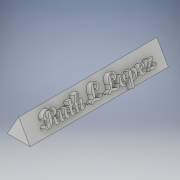
# Autodesk Inventor part: namePlateV01
Saved by Autodesk Inventor 2018.2 (Build 222227000, 227)
## iProperties
Created: 2018-02-15
Part Number: namePlateV01
Material: Generic
Document SubType Name: Modeling
Designer: steele
Density: 1 g/cm^3
Appearance: Default
Author: steele
Autodesk Inventor part; units mm, degrees
ref_plane "YZ Plane" through (0, 0, 0) normal (1, 0, 0) x (0, 1, 0)
ref_plane "XZ Plane" through (0, 0, 0) normal (0, 1, 0) x (-1, 0, 0)
ref_plane "XY Plane" through (0, 0, 0) normal (0, 0, 1) x (1, 0, 0)
sketch "Sketch1" plane through (0, 0, 0) normal (0, 0, 1) x (1, 0, 0)
  line L0 (0, 0) -> (12.7, 0)
  line L1 (0, 0) -> (0, 34.2679) construction
  line L2 (0, 21.997) -> (12.7, 0)
  line L3 (0, 0) -> (-12.7, 0)
  line L4 (0, 21.997) -> (-12.7, 0)
  dimension "d0" = 12.7
  dimension "d1" = 25.4
  constraints: 10 end point, 1 horizontal, 1 point on line, 1 symmetric about line, 1 vertical
  measures "d0" distance of L0.start L0.end
  measures "d1" distance of L2.start L0.end
extrude "Extrusion1" add sketch "Sketch1" along normal mid plane 152.4
sketch "Sketch2" plane through (0, 21.997, 76.2) normal (0.866, 0.5, 0) x (0, 0, -1)
  line L0 (0, -25.4) -> (0, 0) construction
  line L1 (152.4, -12.7) -> (0, -12.7) construction
  line L2 (0, -12.7) -> (152.4, -12.7) construction
  spline S0 degree 2 poles (32.3187, -16.7248) (31.0929, -18.0517) (29.1594, -19.2901) (28.1611, -19.2901) knots 0 0 0 1 2 2 2
  spline S1 degree 2 poles (28.1611, -19.2901) (27.1376, -19.2901) (25.8865, -17.9506) (25.8865, -16.8638) knots 0 0 0 1 2 2 2
  spline S2 degree 2 poles (25.8865, -16.8638) (25.8865, -16.2067) (26.4804, -13.9321) (26.4804, -13.3255) knots 0 0 0 1 2 2 2
  spline S3 degree 2 poles (26.4804, -13.3255) (26.4804, -12.3399) (25.8486, -12.3146) knots 0 0 0 1 1 1
  spline S4 degree 2 poles (25.8486, -12.3146) (25.4569, -12.2893) (25.4569, -11.9481) knots 0 0 0 1 1 1
  spline S5 degree 2 poles (25.4569, -11.9481) (25.4569, -11.3289) (25.9118, -11.3289) knots 0 0 0 1 1 1
  line L3 (25.9118, -11.3289) -> (26.6068, -11.3668)
  spline S6 degree 2 poles (26.6068, -11.3668) (27.6051, -11.3668) (28.7677, -9.4334) (28.7677, -8.0686) knots 0 0 0 1 2 2 2
  spline S7 degree 2 poles (28.7677, -8.0686) (28.7677, -4.8968) (25.1536, -4.8968) knots 0 0 0 1 1 1
  spline S8 degree 2 poles (25.1536, -4.8968) (22.8537, -4.8968) (19.2901, -7.3862) (19.2901, -8.9153) knots 0 0 0 1 2 2 2
  spline S9 degree 2 poles (19.2901, -8.9153) (19.2901, -9.7746) (20.1494, -10.2169) knots 0 0 0 1 1 1
  spline S10 degree 2 poles (20.1494, -10.2169) (20.5538, -10.4317) (20.5538, -10.735) knots 0 0 0 1 1 1
  spline S11 degree 2 poles (20.5538, -10.735) (20.5538, -11.0003) (18.9615, -11.708) (18.6709, -11.708) knots 0 0 0 1 2 2 2
  spline S12 degree 2 poles (18.6709, -11.708) (18.2033, -11.708) (17.4578, -10.5075) (17.4578, -9.724) knots 0 0 0 1 2 2 2
  spline S13 degree 2 poles (17.4578, -9.724) (17.4578, -7.3989) (22.1839, -4.088) (25.5832, -4.088) knots 0 0 0 1 2 2 2
  spline S14 degree 2 poles (25.5832, -4.088) (28.4391, -4.088) (31.6236, -6.5396) (31.6236, -8.2961) knots 0 0 0 1 2 2 2
  spline S15 degree 2 poles (31.6236, -8.2961) (31.6236, -9.3955) (29.8671, -11.4679) (27.3018, -12.0492) knots 0 0 0 1 2 2 2
  spline S16 degree 2 poles (27.3018, -12.0492) (28.237, -12.58) (29.0836, -13.831) (29.0836, -14.7788) knots 0 0 0 1 2 2 2
  spline S17 degree 2 poles (29.0836, -14.7788) (29.0836, -15.2969) (28.8688, -16.5985) (28.8688, -16.7754) knots 0 0 0 1 2 2 2
  spline S18 degree 2 poles (28.8688, -16.7754) (28.8688, -17.6726) (29.5891, -17.6726) knots 0 0 0 1 1 1
  spline S19 degree 2 poles (29.5891, -17.6726) (30.5369, -17.6726) (32.3187, -15.5117) knots 0 0 0 1 1 1
  line L4 (32.3187, -15.5117) -> (32.3187, -16.7248)
  spline S20 degree 2 poles (26.9227, -6.7038) (26.0634, -7.3989) (25.4821, -8.9911) (24.8882, -13.2623) (24.1426, -15.7897) (22.2977, -18.0264) (19.6818, -19.2901) (18.2791, -19.2901) knots 0 0 0 1 2 3 4 5 6 6 6
  spline S21 degree 2 poles (18.2791, -19.2901) (16.7754, -19.2901) (15.2716, -17.8242) (15.2716, -16.8765) knots 0 0 0 1 2 2 2
  spline S22 degree 2 poles (15.2716, -16.8765) (15.2716, -16.5732) (15.7391, -16.0803) (17.205, -15.2463) (17.483, -15.2463) knots 0 0 0 1 2 3 3 3
  spline S23 degree 2 poles (17.483, -15.2463) (17.8242, -15.2463) (17.8242, -15.6507) knots 0 0 0 1 1 1
  spline S24 degree 2 poles (17.8242, -15.6507) (17.8242, -15.7392) (17.6094, -16.9776) (17.6094, -17.1039) knots 0 0 0 1 2 2 2
  spline S25 degree 2 poles (17.6094, -17.1039) (17.6094, -17.6852) (18.2791, -18.4561) (18.7973, -18.4561) knots 0 0 0 1 2 2 2
  spline S26 degree 2 poles (18.7973, -18.4561) (19.884, -18.4561) (21.5647, -15.6886) (22.2471, -10.28) (23.3591, -7.8411) (25.4948, -6.35) (26.3414, -6.35) knots 0 0 0 1 2 3 4 5 5 5
  spline S27 degree 2 poles (26.3414, -6.35) (26.5815, -6.35) (26.9227, -6.7038) knots 0 0 0 1 1 1
  spline S28 degree 2 poles (43.5149, -16.7375) (42.1248, -18.0391) (40.2672, -19.2901) (39.5216, -19.2901) knots 0 0 0 1 2 2 2
  spline S29 degree 2 poles (39.5216, -19.2901) (38.6876, -19.2901) (37.803, -17.9632) (37.803, -16.8386) knots 0 0 0 1 2 2 2
  spline S30 degree 2 poles (37.803, -16.8386) (36.6404, -18.1022) (34.8207, -19.3154) (33.9488, -19.3154) knots 0 0 0 1 2 2 2
  spline S31 degree 2 poles (33.9488, -19.3154) (33.14, -19.3154) (32.1796, -17.9885) (32.1796, -16.8638) knots 0 0 0 1 2 2 2
  spline S32 degree 2 poles (32.1796, -16.8638) (32.1796, -14.6777) (33.6455, -10.7097) knots 0 0 0 1 1 1
  line L5 (33.6455, -10.7097) -> (36.4635, -10.1537)
  spline S33 degree 2 poles (36.4635, -10.1537) (34.7196, -15.1831) (34.7196, -16.6111) knots 0 0 0 1 1 1
  spline S34 degree 2 poles (34.7196, -16.6111) (34.7196, -17.6094) (35.4779, -17.6094) knots 0 0 0 1 1 1
  spline S35 degree 2 poles (35.4779, -17.6094) (36.0212, -17.6094) (37.6388, -15.8402) (37.8409, -15.1831) knots 0 0 0 1 2 2 2
  line L6 (37.8409, -15.1831) -> (39.2184, -10.7097)
  line L7 (39.2184, -10.7097) -> (42.0869, -10.1284)
  spline S36 degree 2 poles (42.0869, -10.1284) (41.0886, -13.2876) (40.343, -15.8529) (40.343, -16.3584) knots 0 0 0 1 2 2 2
  spline S37 degree 2 poles (40.343, -16.3584) (40.343, -17.344) (41.0128, -17.344) knots 0 0 0 1 1 1
  spline S38 degree 2 poles (41.0128, -17.344) (41.5688, -17.344) (42.6303, -16.3457) knots 0 0 0 1 1 1
  line L8 (42.6303, -16.3457) -> (43.5149, -15.5243)
  line L9 (43.5149, -15.5243) -> (43.5149, -16.7375)
  spline S39 degree 2 poles (49.6943, -16.7375) (48.3674, -18.0391) (46.434, -19.2901) (45.562, -19.2901) knots 0 0 0 1 2 2 2
  spline S40 degree 2 poles (45.562, -19.2901) (44.6648, -19.2901) (43.5401, -17.7737) (43.5401, -16.5353) knots 0 0 0 1 2 2 2
  spline S41 degree 2 poles (43.5401, -16.5353) (43.5401, -15.4359) (44.0835, -13.6541) knots 0 0 0 1 1 1
  line L10 (44.0835, -13.6541) -> (44.5258, -12.0618)
  line L11 (44.5258, -12.0618) -> (43.7171, -12.0998)
  line L12 (43.7171, -12.0998) -> (44.0583, -10.457)
  line L13 (44.0583, -10.457) -> (45.0566, -10.4191)
  line L14 (45.0566, -10.4191) -> (46.0422, -7.1461)
  line L15 (46.0422, -7.1461) -> (48.8476, -6.5648)
  line L16 (48.8476, -6.5648) -> (47.7608, -10.2169)
  line L17 (47.7608, -10.2169) -> (49.2393, -10.1284)
  line L18 (49.2393, -10.1284) -> (48.8982, -11.7459)
  line L19 (48.8982, -11.7459) -> (47.268, -11.8723)
  line L20 (47.268, -11.8723) -> (46.5603, -14.2227)
  spline S42 degree 2 poles (46.5603, -14.2227) (46.2065, -15.4485) (46.2065, -16.1688) knots 0 0 0 1 1 1
  spline S43 degree 2 poles (46.2065, -16.1688) (46.2065, -16.6616) (46.6993, -17.2808) (47.0911, -17.2808) knots 0 0 0 1 2 2 2
  spline S44 degree 2 poles (47.0911, -17.2808) (47.6218, -17.2808) (48.6707, -16.5985) (49.6943, -15.5243) knots 0 0 0 1 2 2 2
  line L21 (49.6943, -15.5243) -> (49.6943, -16.7375)
  spline S45 degree 2 poles (60.107, -16.7375) (57.6176, -19.3154) (56.0127, -19.3154) knots 0 0 0 1 1 1
  spline S46 degree 2 poles (56.0127, -19.3154) (55.305, -19.3154) (54.3699, -18.3423) (54.3699, -17.5968) knots 0 0 0 1 2 2 2
  spline S47 degree 2 poles (54.3699, -17.5968) (54.3699, -16.3331) (55.3303, -14.0458) knots 0 0 0 1 1 1
  spline S48 degree 2 poles (55.3303, -14.0458) (55.8484, -12.8074) (55.8484, -12.4283) knots 0 0 0 1 1 1
  spline S49 degree 2 poles (55.8484, -12.4283) (55.8484, -11.9987) (55.444, -11.9987) knots 0 0 0 1 1 1
  spline S50 degree 2 poles (55.444, -11.9987) (55.0144, -11.9987) (53.4221, -13.136) (52.5376, -14.1216) knots 0 0 0 1 2 2 2
  spline S51 degree 2 poles (52.5376, -14.1216) (52.1711, -16.0551) (52.1711, -18.772) knots 0 0 0 1 1 1
  line L22 (52.1711, -18.772) -> (49.8333, -19.3154)
  spline S52 degree 2 poles (49.8333, -19.3154) (49.6943, -18.216) (49.6943, -16.927) knots 0 0 0 1 1 1
  spline S53 degree 2 poles (49.6943, -16.927) (49.6943, -13.7931) (51.4129, -8.3972) (53.2579, -5.377) knots 0 0 0 1 2 2 2
  spline S54 degree 2 poles (53.2579, -5.377) (54.6353, -4.8209) (56.6824, -4.1133) (56.8214, -4.1133) knots 0 0 0 1 2 2 2
  spline S55 degree 2 poles (56.8214, -4.1133) (57.0994, -4.1133) (57.4786, -4.9979) (57.4786, -5.655) knots 0 0 0 1 2 2 2
  spline S56 degree 2 poles (57.4786, -5.655) (57.4786, -6.767) (56.1138, -9.4713) (54.6605, -11.3795) knots 0 0 0 1 2 2 2
  spline S57 degree 2 poles (54.6605, -11.3795) (56.0632, -10.5707) (56.9857, -10.1537) (57.4786, -10.1537) knots 0 0 0 1 2 2 2
  spline S58 degree 2 poles (57.4786, -10.1537) (58.0093, -10.1537) (58.6791, -10.9245) (58.6791, -11.5564) knots 0 0 0 1 2 2 2
  spline S59 degree 2 poles (58.6791, -11.5564) (58.6791, -12.5041) (57.1626, -16.4595) (57.1626, -16.9649) knots 0 0 0 1 2 2 2
  spline S60 degree 2 poles (57.1626, -16.9649) (57.1626, -17.1924) (57.4406, -17.5462) (57.6302, -17.5462) knots 0 0 0 1 2 2 2
  spline S61 degree 2 poles (57.6302, -17.5462) (58.2999, -17.5462) (60.107, -15.5243) knots 0 0 0 1 1 1
  line L23 (60.107, -15.5243) -> (60.107, -16.7375)
  spline S62 degree 2 poles (52.8282, -12.4283) (56.5813, -8.0686) (56.5813, -6.0088) knots 0 0 0 1 1 1
  spline S63 degree 2 poles (56.5813, -6.0088) (56.5813, -5.377) (56.2401, -5.377) knots 0 0 0 1 1 1
  spline S64 degree 2 poles (56.2401, -5.377) (55.6589, -5.377) (53.5106, -9.5092) (52.8282, -12.4283) knots 0 0 0 1 2 2 2
  spline S65 degree 2 poles (79.2392, -16.7248) (76.7497, -19.2522) (74.1465, -19.2522) knots 0 0 0 1 1 1
  spline S66 degree 2 poles (74.1465, -19.2522) (73.3883, -19.2522) (71.9983, -18.8604) (69.989, -17.9506) (69.2308, -17.7358) knots 0 0 0 1 2 3 3 3
  spline S67 degree 2 poles (69.2308, -17.7358) (67.8155, -19.2901) (66.6655, -19.2901) knots 0 0 0 1 1 1
  spline S68 degree 2 poles (66.6655, -19.2901) (66.2738, -19.2901) (65.743, -18.7594) (65.743, -18.3929) knots 0 0 0 1 2 2 2
  spline S69 degree 2 poles (65.743, -18.3929) (65.743, -17.5968) (67.31, -16.3836) (68.738, -16.1562) knots 0 0 0 1 2 2 2
  spline S70 degree 2 poles (68.738, -16.1562) (69.3319, -15.3348) (69.6731, -13.7678) (69.7615, -11.9734) knots 0 0 0 1 2 2 2
  spline S71 degree 2 poles (69.7615, -11.9734) (69.9385, -8.2834) (73.5399, -4.088) (75.6503, -4.088) knots 0 0 0 1 2 2 2
  spline S72 degree 2 poles (75.6503, -4.088) (77.1035, -4.088) (78.9611, -5.9203) (78.9611, -7.3483) knots 0 0 0 1 2 2 2
  spline S73 degree 2 poles (78.9611, -7.3483) (78.9611, -9.0037) (77.0151, -11.4805) (75.7388, -11.4805) knots 0 0 0 1 2 2 2
  spline S74 degree 2 poles (75.7388, -11.4805) (75.0816, -11.4805) (74.3234, -10.7602) (74.3234, -10.1284) knots 0 0 0 1 2 2 2
  spline S75 degree 2 poles (74.3234, -10.1284) (74.3234, -9.7999) (74.4498, -9.3702) knots 0 0 0 1 1 1
  spline S76 degree 2 poles (74.4498, -9.3702) (74.7278, -9.6988) (75.1701, -9.6988) knots 0 0 0 1 1 1
  spline S77 degree 2 poles (75.1701, -9.6988) (75.8778, -9.6988) (76.9519, -7.9928) (76.9519, -6.8176) knots 0 0 0 1 2 2 2
  spline S78 degree 2 poles (76.9519, -6.8176) (76.9519, -5.9077) (76.1305, -4.8715) (75.4102, -4.8715) knots 0 0 0 1 2 2 2
  spline S79 degree 2 poles (75.4102, -4.8715) (74.5509, -4.8715) (73.5905, -6.1099) (73.2114, -7.8411) (72.7944, -11.6827) (71.7961, -14.6524) (70.4187, -16.0803) knots 0 0 0 1 2 3 4 5 5 5
  spline S80 degree 2 poles (70.4187, -16.0803) (71.3159, -16.0172) (72.6301, -16.3457) (75.069, -17.2808) (75.9536, -17.2808) knots 0 0 0 1 2 3 3 3
  spline S81 degree 2 poles (75.9536, -17.2808) (77.6722, -17.2808) (79.2392, -15.5117) knots 0 0 0 1 1 1
  line L24 (79.2392, -15.5117) -> (79.2392, -16.7248)
  spline S82 degree 2 poles (98.2576, -16.7248) (95.7681, -19.2522) (93.1649, -19.2522) knots 0 0 0 1 1 1
  spline S83 degree 2 poles (93.1649, -19.2522) (92.4067, -19.2522) (91.0167, -18.8604) (89.0074, -17.9506) (88.2492, -17.7358) knots 0 0 0 1 2 3 3 3
  spline S84 degree 2 poles (88.2492, -17.7358) (86.8339, -19.2901) (85.6839, -19.2901) knots 0 0 0 1 1 1
  spline S85 degree 2 poles (85.6839, -19.2901) (85.2922, -19.2901) (84.7614, -18.7594) (84.7614, -18.3929) knots 0 0 0 1 2 2 2
  spline S86 degree 2 poles (84.7614, -18.3929) (84.7614, -17.5968) (86.3284, -16.3836) (87.7564, -16.1562) knots 0 0 0 1 2 2 2
  spline S87 degree 2 poles (87.7564, -16.1562) (88.3503, -15.3348) (88.6915, -13.7678) (88.7799, -11.9734) knots 0 0 0 1 2 2 2
  spline S88 degree 2 poles (88.7799, -11.9734) (88.9569, -8.2834) (92.5584, -4.088) (94.6687, -4.088) knots 0 0 0 1 2 2 2
  spline S89 degree 2 poles (94.6687, -4.088) (96.1219, -4.088) (97.9796, -5.9203) (97.9796, -7.3483) knots 0 0 0 1 2 2 2
  spline S90 degree 2 poles (97.9796, -7.3483) (97.9796, -9.0037) (96.0335, -11.4805) (94.7572, -11.4805) knots 0 0 0 1 2 2 2
  spline S91 degree 2 poles (94.7572, -11.4805) (94.1, -11.4805) (93.3418, -10.7602) (93.3418, -10.1284) knots 0 0 0 1 2 2 2
  spline S92 degree 2 poles (93.3418, -10.1284) (93.3418, -9.7999) (93.4682, -9.3702) knots 0 0 0 1 1 1
  spline S93 degree 2 poles (93.4682, -9.3702) (93.7462, -9.6988) (94.1885, -9.6988) knots 0 0 0 1 1 1
  spline S94 degree 2 poles (94.1885, -9.6988) (94.8962, -9.6988) (95.9703, -7.9928) (95.9703, -6.8176) knots 0 0 0 1 2 2 2
  spline S95 degree 2 poles (95.9703, -6.8176) (95.9703, -5.9077) (95.1489, -4.8715) (94.4286, -4.8715) knots 0 0 0 1 2 2 2
  spline S96 degree 2 poles (94.4286, -4.8715) (93.5693, -4.8715) (92.6089, -6.1099) (92.2298, -7.8411) (91.8128, -11.6827) (90.8145, -14.6524) (89.4371, -16.0803) knots 0 0 0 1 2 3 4 5 5 5
  spline S97 degree 2 poles (89.4371, -16.0803) (90.3343, -16.0172) (91.6485, -16.3457) (94.0874, -17.2808) (94.972, -17.2808) knots 0 0 0 1 2 3 3 3
  spline S98 degree 2 poles (94.972, -17.2808) (96.6906, -17.2808) (98.2576, -15.5117) knots 0 0 0 1 1 1
  line L25 (98.2576, -15.5117) -> (98.2576, -16.7248)
  spline S99 degree 2 poles (107.672, -16.7375) (107.1412, -17.205) (106.1303, -17.5841) (105.8397, -17.5841) knots 0 0 0 1 2 2 2
  spline S100 degree 2 poles (105.8397, -17.5841) (105.0814, -17.5841) (104.3359, -17.0028) knots 0 0 0 1 1 1
  spline S101 degree 2 poles (104.3359, -17.0028) (102.8195, -19.2901) (100.8734, -19.2901) knots 0 0 0 1 1 1
  spline S102 degree 2 poles (100.8734, -19.2901) (99.6602, -19.2901) (98.1438, -17.4578) (98.1438, -15.954) knots 0 0 0 1 2 2 2
  spline S103 degree 2 poles (98.1438, -15.954) (98.1438, -13.5656) (101.5431, -10.1284) (103.9062, -10.1284) knots 0 0 0 1 2 2 2
  spline S104 degree 2 poles (103.9062, -10.1284) (104.7908, -10.1284) (105.6248, -10.5201) (105.8144, -11.0383) (105.8144, -11.4426) knots 0 0 0 1 2 3 3 3
  spline S105 degree 2 poles (105.8144, -11.4426) (105.8144, -13.4013) (104.7402, -16.2573) knots 0 0 0 1 1 1
  spline S106 degree 2 poles (104.7402, -16.2573) (105.2836, -16.7501) (105.8649, -16.7501) knots 0 0 0 1 1 1
  spline S107 degree 2 poles (105.8649, -16.7501) (106.5726, -16.7501) (107.672, -15.5243) knots 0 0 0 1 1 1
  line L26 (107.672, -15.5243) -> (107.672, -16.7375)
  spline S108 degree 2 poles (104.2095, -10.8613) (104.0452, -10.7982) (103.7546, -10.7982) knots 0 0 0 1 1 1
  spline S109 degree 2 poles (103.7546, -10.7982) (102.3898, -10.7982) (100.8481, -13.6541) (100.8481, -15.5622) knots 0 0 0 1 2 2 2
  spline S110 degree 2 poles (100.8481, -15.5622) (100.8481, -16.6237) (101.5179, -17.799) (102.1244, -17.799) knots 0 0 0 1 2 2 2
  spline S111 degree 2 poles (102.1244, -17.799) (102.87, -17.799) (103.7419, -16.4215) knots 0 0 0 1 1 1
  spline S112 degree 2 poles (103.7419, -16.4215) (102.7436, -15.1831) (102.7436, -13.7552) knots 0 0 0 1 1 1
  spline S113 degree 2 poles (102.7436, -13.7552) (102.7436, -12.0745) (104.2095, -10.8613) knots 0 0 0 1 1 1
  spline S114 degree 2 poles (112.8025, -11.9355) (113.5481, -11.0256) (114.9003, -10.1537) (115.7216, -10.1537) knots 0 0 0 1 2 2 2
  spline S115 degree 2 poles (115.7216, -10.1537) (116.7705, -10.1537) (118.11, -11.7838) (118.11, -13.0981) knots 0 0 0 1 2 2 2
  spline S116 degree 2 poles (118.11, -13.0981) (118.11, -15.4232) (114.9129, -19.2901) (113.03, -19.2901) knots 0 0 0 1 2 2 2
  spline S117 degree 2 poles (113.03, -19.2901) (112.5119, -19.2901) (111.8927, -19.0626) (111.3999, -18.6456) knots 0 0 0 1 2 2 2
  spline S118 degree 2 poles (111.3999, -18.6456) (110.6416, -21.9691) (110.4268, -23.9784) knots 0 0 0 1 1 1
  line L27 (110.4268, -23.9784) -> (107.7604, -24.4459)
  spline S119 degree 2 poles (107.7604, -24.4459) (108.506, -19.5302) (109.656, -14.5007) knots 0 0 0 1 1 1
  spline S120 degree 2 poles (109.656, -14.5007) (108.2659, -16.3078) (107.7857, -16.7375) knots 0 0 0 1 1 1
  line L28 (107.7857, -16.7375) -> (107.5456, -16.7375)
  line L29 (107.5456, -16.7375) -> (107.5456, -15.7897)
  spline S121 degree 2 poles (107.5456, -15.7897) (109.5422, -13.6414) (110.8312, -10.5581) knots 0 0 0 1 1 1
  line L30 (110.8312, -10.5581) -> (113.1943, -10.1284)
  line L31 (113.1943, -10.1284) -> (112.8025, -11.9355)
  spline S122 degree 2 poles (111.602, -17.5462) (112.1454, -18.4561) (112.8025, -18.4561) knots 0 0 0 1 1 1
  spline S123 degree 2 poles (112.8025, -18.4561) (113.864, -18.4561) (115.4815, -15.2337) (115.4815, -13.7046) knots 0 0 0 1 2 2 2
  spline S124 degree 2 poles (115.4815, -13.7046) (115.4815, -12.8959) (114.8244, -11.8976) (114.2937, -11.8976) knots 0 0 0 1 2 2 2
  spline S125 degree 2 poles (114.2937, -11.8976) (113.8893, -11.8976) (112.9921, -12.6305) (112.5245, -13.6035) (112.2339, -14.8167) knots 0 0 0 1 2 3 3 3
  line L32 (112.2339, -14.8167) -> (111.602, -17.5462)
  spline S126 degree 2 poles (127.7266, -16.7375) (126.3998, -18.0391) (124.2768, -19.2901) (123.0005, -19.2901) knots 0 0 0 1 2 2 2
  spline S127 degree 2 poles (123.0005, -19.2901) (121.5725, -19.2901) (119.816, -17.4704) (119.816, -15.9793) knots 0 0 0 1 2 2 2
  spline S128 degree 2 poles (119.816, -15.9793) (119.816, -13.7552) (122.8994, -10.1537) (124.7822, -10.1537) knots 0 0 0 1 2 2 2
  spline S129 degree 2 poles (124.7822, -10.1537) (125.7553, -10.1537) (126.9305, -11.1646) (126.9305, -11.9734) knots 0 0 0 1 2 2 2
  spline S130 degree 2 poles (126.9305, -11.9734) (126.9305, -14.1469) (122.3181, -15.4991) knots 0 0 0 1 1 1
  spline S131 degree 2 poles (122.3181, -15.4991) (122.7351, -17.5462) (124.5042, -17.5462) knots 0 0 0 1 1 1
  spline S132 degree 2 poles (124.5042, -17.5462) (125.1993, -17.5462) (126.4629, -16.8006) (127.7266, -15.5243) knots 0 0 0 1 2 2 2
  line L33 (127.7266, -15.5243) -> (127.7266, -16.7375)
  spline S133 degree 2 poles (122.2296, -14.7914) (124.9212, -14.0332) (124.9212, -11.9987) knots 0 0 0 1 1 1
  spline S134 degree 2 poles (124.9212, -11.9987) (124.9212, -10.9877) (124.1883, -10.9877) knots 0 0 0 1 1 1
  spline S135 degree 2 poles (124.1883, -10.9877) (123.4933, -10.9877) (122.2296, -13.0981) (122.2296, -14.7914) knots 0 0 0 1 2 2 2
  spline S136 degree 2 poles (138.1014, -16.7375) (136.6735, -18.3044) (135.2329, -19.3154) (134.5379, -19.3154) knots 0 0 0 1 2 2 2
  spline S137 degree 2 poles (134.5379, -19.3154) (134.1335, -19.3154) (132.0105, -18.6203) (131.4671, -18.6203) knots 0 0 0 1 2 2 2
  spline S138 degree 2 poles (131.4671, -18.6203) (130.7847, -18.6203) (130.1655, -19.3154) (130.0644, -19.3154) knots 0 0 0 1 2 2 2
  spline S139 degree 2 poles (130.0644, -19.3154) (129.5463, -19.3154) (129.3315, -19.2775) (129.3315, -19.2269) knots 0 0 0 1 2 2 2
  spline S140 degree 2 poles (129.3315, -19.2269) (129.3315, -18.9868) (131.1259, -16.788) knots 0 0 0 1 1 1
  line L34 (131.1259, -16.788) -> (134.7527, -12.3778)
  spline S141 degree 2 poles (134.7527, -12.3778) (134.1335, -12.5041) (133.4385, -12.5041) knots 0 0 0 1 1 1
  spline S142 degree 2 poles (133.4385, -12.5041) (132.4907, -12.5041) (131.4798, -12.1882) knots 0 0 0 1 1 1
  spline S143 degree 2 poles (131.4798, -12.1882) (129.5842, -14.9051) (127.8024, -16.7375) knots 0 0 0 1 1 1
  line L35 (127.8024, -16.7375) -> (127.5623, -16.7375)
  line L36 (127.5623, -16.7375) -> (127.5623, -15.7897)
  spline S144 degree 2 poles (127.5623, -15.7897) (128.8892, -14.4249) (131.366, -11.0383) (131.7578, -10.1537) (131.8841, -10.1537) knots 0 0 0 1 2 3 3 3
  spline S145 degree 2 poles (131.8841, -10.1537) (131.96, -10.1537) (133.7417, -10.4317) (134.2978, -10.4317) knots 0 0 0 1 2 2 2
  spline S146 degree 2 poles (134.2978, -10.4317) (135.2834, -10.4317) (136.9262, -10.1537) (137.0652, -10.1537) knots 0 0 0 1 2 2 2
  spline S147 degree 2 poles (137.0652, -10.1537) (137.2674, -10.1537) (137.2674, -10.2548) knots 0 0 0 1 1 1
  spline S148 degree 2 poles (137.2674, -10.2548) (137.2548, -10.6339) (135.5614, -12.6558) knots 0 0 0 1 1 1
  line L37 (135.5614, -12.6558) -> (132.1874, -16.7627)
  spline S149 degree 2 poles (132.1874, -16.7627) (132.6044, -16.7248) (132.8698, -16.7248) knots 0 0 0 1 1 1
  spline S150 degree 2 poles (132.8698, -16.7248) (133.072, -16.7248) (135.3972, -17.205) (135.6246, -17.205) knots 0 0 0 1 2 2 2
  spline S151 degree 2 poles (135.6246, -17.205) (136.2817, -17.205) (137.2042, -16.4974) (138.1014, -15.5243) knots 0 0 0 1 2 2 2
  line L38 (138.1014, -15.5243) -> (138.1014, -16.7375)
  point P0 (76.2, -19.05)
  constraints: 2 end point, 2 horizontal, 1 midpoint
extrude "Extrusion2" add sketch "Sketch2" along normal blind 6.35
body "Solid1"
